Autodesk Fusion 360 part; units mm, degrees
note: some values were not read from the file. Set by a fixed rule: the direction of a hole.
(part 7 of 10)
  arc A53 (93.84, 10.795) -> (97.04, 10.795) centre (95.44, 10.795) ccw
  arc A54 (97.04, 15.875) -> (93.84, 15.875) centre (95.44, 15.875) ccw
  arc A55 (93.84, 15.875) -> (97.04, 15.875) centre (95.44, 15.875) ccw
  arc A56 (6.731, 3.81) -> (0.889, 3.81) centre (3.81, 3.81) ccw
  arc A57 (0.889, 3.81) -> (6.731, 3.81) centre (3.81, 3.81) ccw
  arc A58 (2.31, 3.81) -> (5.31, 3.81) centre (3.81, 3.81) ccw
  arc A59 (5.31, 3.81) -> (2.31, 3.81) centre (3.81, 3.81) ccw
  arc A60 (99.441, 76.2) -> (93.599, 76.2) centre (96.52, 76.2) ccw
  arc A61 (93.599, 76.2) -> (99.441, 76.2) centre (96.52, 76.2) ccw
  arc A62 (95.02, 76.2) -> (98.02, 76.2) centre (96.52, 76.2) ccw
  arc A63 (98.02, 76.2) -> (95.02, 76.2) centre (96.52, 76.2) ccw
  arc A64 (0.889, 76.2) -> (6.731, 76.2) centre (3.81, 76.2) ccw
  arc A65 (6.731, 76.2) -> (0.889, 76.2) centre (3.81, 76.2) ccw
  arc A66 (5.31, 76.2) -> (2.31, 76.2) centre (3.81, 76.2) ccw
  arc A67 (2.31, 76.2) -> (5.31, 76.2) centre (3.81, 76.2) ccw
  arc A68 (99.441, 3.81) -> (93.599, 3.81) centre (96.52, 3.81) ccw
  arc A69 (93.599, 3.81) -> (99.441, 3.81) centre (96.52, 3.81) ccw
  arc A70 (98.02, 3.81) -> (95.02, 3.81) centre (96.52, 3.81) ccw
  arc A71 (95.02, 3.81) -> (98.02, 3.81) centre (96.52, 3.81) ccw
  line L5675 (36.52, 58.32) -> (36.52, 71.07)
  line L5676 (36.52, 71.07) -> (4.02, 71.07)
  line L5677 (4.02, 71.07) -> (4.02, 58.32)
  line L5678 (4.02, 58.32) -> (36.52, 58.32)
  line L5679 (63.81, 71.22) -> (63.81, 58.47)
  line L5680 (63.81, 58.47) -> (96.31, 58.47)
  line L5681 (96.31, 58.47) -> (96.31, 71.22)
  line L5682 (96.31, 71.22) -> (63.81, 71.22)
  line L5683 (10.143, 54.229) -> (1.143, 54.229)
  line L5684 (1.143, 54.229) -> (1.143, 32.229)
  line L5685 (1.143, 32.229) -> (10.143, 32.229)
  line L5686 (10.143, 32.229) -> (10.143, 54.229)
  line L5687 (22.843, 54.229) -> (13.843, 54.229)
  line L5688 (13.843, 54.229) -> (13.843, 32.229)
  line L5689 (13.843, 32.229) -> (22.843, 32.229)
  line L5690 (22.843, 32.229) -> (22.843, 54.229)
  line L5691 (35.543, 54.229) -> (26.543, 54.229)
  line L5692 (26.543, 54.229) -> (26.543, 32.229)
  line L5693 (26.543, 32.229) -> (35.543, 32.229)
  line L5694 (35.543, 32.229) -> (35.543, 54.229)
  line L5695 (48.243, 54.229) -> (39.243, 54.229)
  line L5696 (39.243, 54.229) -> (39.243, 32.229)
  line L5697 (39.243, 32.229) -> (48.243, 32.229)
  line L5698 (48.243, 32.229) -> (48.243, 54.229)
  line L5699 (61.578, 54.229) -> (52.578, 54.229)
  line L5700 (52.578, 54.229) -> (52.578, 32.229)
  line L5701 (52.578, 32.229) -> (61.578, 32.229)
  line L5702 (61.578, 32.229) -> (61.578, 54.229)
  line L5703 (74.278, 54.229) -> (65.278, 54.229)
  line L5704 (65.278, 54.229) -> (65.278, 32.229)
  line L5705 (65.278, 32.229) -> (74.278, 32.229)
  line L5706 (74.278, 32.229) -> (74.278, 54.229)
  line L5707 (86.978, 54.229) -> (77.978, 54.229)
  line L5708 (77.978, 54.229) -> (77.978, 32.229)
  line L5709 (77.978, 32.229) -> (86.978, 32.229)
  line L5710 (86.978, 32.229) -> (86.978, 54.229)
  line L5711 (99.043, 54.229) -> (90.043, 54.229)
  line L5712 (90.043, 54.229) -> (90.043, 32.229)
  line L5713 (90.043, 32.229) -> (99.043, 32.229)
  line L5714 (99.043, 32.229) -> (99.043, 54.229)
  line L5715 (50.8, 79.375) -> (50.8, 71.375)
  line L5716 (55.88, 79.375) -> (50.8, 79.375)
  line L5717 (50.8, 79.375) -> (45.72, 79.375)
  line L5718 (45.72, 79.375) -> (45.72, 78.74)
  line L5719 (45.72, 78.74) -> (45.72, 72.0725)
  line L5720 (45.72, 72.0725) -> (45.72, 71.375)
  line L5721 (45.72, 71.375) -> (50.8, 71.375)
  line L5722 (50.8, 71.375) -> (55.88, 71.375)
  line L5723 (55.88, 71.375) -> (55.88, 72.0725)
  line L5724 (55.88, 72.0725) -> (55.88, 72.263)
  line L5725 (55.88, 72.263) -> (55.88, 73.025)
  line L5726 (55.88, 73.025) -> (55.88, 78.74)
  line L5727 (55.88, 78.74) -> (55.88, 79.375)
  line L5728 (55.88, 72.0725) -> (45.72, 72.0725)
  line L5729 (55.88, 72.263) -> (56.388, 71.755)
  line L5730 (56.388, 71.755) -> (56.388, 73.533)
  line L5731 (56.388, 73.533) -> (55.88, 73.025)
  line L5732 (55.88, 78.74) -> (45.72, 78.74)
  line L5733 (0.635, 13.335) -> (8.635, 13.335)
  line L5734 (0.635, 18.415) -> (0.635, 13.335)
  line L5735 (0.635, 13.335) -> (0.635, 8.255)
  line L5736 (0.635, 8.255) -> (1.27, 8.255)
  line L5737 (1.27, 8.255) -> (7.9375, 8.255)
  line L5738 (7.9375, 8.255) -> (8.635, 8.255)
  line L5739 (8.635, 8.255) -> (8.635, 13.335)
  line L5740 (8.635, 13.335) -> (8.635, 18.415)
  line L5741 (8.635, 18.415) -> (7.9375, 18.415)
  line L5742 (7.9375, 18.415) -> (7.747, 18.415)
  line L5743 (7.747, 18.415) -> (6.985, 18.415)
  line L5744 (6.985, 18.415) -> (1.27, 18.415)
  line L5745 (1.27, 18.415) -> (0.635, 18.415)
  line L5746 (7.9375, 18.415) -> (7.9375, 8.255)
  line L5747 (7.747, 18.415) -> (8.255, 18.923)
  line L5748 (8.255, 18.923) -> (6.477, 18.923)
  line L5749 (6.477, 18.923) -> (6.985, 18.415)
  line L5750 (1.27, 18.415) -> (1.27, 8.255)
  line L5751 (18.415, 8.89) -> (18.415, 0.89)
  line L5752 (23.495, 8.89) -> (18.415, 8.89)
  line L5753 (18.415, 8.89) -> (13.335, 8.89)
  line L5754 (13.335, 8.89) -> (13.335, 8.255)
  line L5755 (13.335, 8.255) -> (13.335, 1.5875)
  line L5756 (13.335, 1.5875) -> (13.335, 0.89)
  line L5757 (13.335, 0.89) -> (18.415, 0.89)
  line L5758 (18.415, 0.89) -> (23.495, 0.89)
  line L5759 (23.495, 0.89) -> (23.495, 1.5875)
  line L5760 (23.495, 1.5875) -> (23.495, 1.778)
  line L5761 (23.495, 1.778) -> (23.495, 2.54)
  line L5762 (23.495, 2.54) -> (23.495, 8.255)
  line L5763 (23.495, 8.255) -> (23.495, 8.89)
  line L5764 (23.495, 1.5875) -> (13.335, 1.5875)
  line L5765 (23.495, 1.778) -> (24.003, 1.27)
  line L5766 (24.003, 1.27) -> (24.003, 3.048)
  line L5767 (24.003, 3.048) -> (23.495, 2.54)
  line L5768 (23.495, 8.255) -> (13.335, 8.255)
  line L5769 (31.115, 8.89) -> (31.115, 0.89)
  line L5770 (36.195, 8.89) -> (31.115, 8.89)
  line L5771 (31.115, 8.89) -> (26.035, 8.89)
  line L5772 (26.035, 8.89) -> (26.035, 8.255)
  line L5773 (26.035, 8.255) -> (26.035, 1.5875)
  line L5774 (26.035, 1.5875) -> (26.035, 0.89)
  line L5775 (26.035, 0.89) -> (31.115, 0.89)
  line L5776 (31.115, 0.89) -> (36.195, 0.89)
  line L5777 (36.195, 0.89) -> (36.195, 1.5875)
  line L5778 (36.195, 1.5875) -> (36.195, 1.778)
  line L5779 (36.195, 1.778) -> (36.195, 2.54)
  line L5780 (36.195, 2.54) -> (36.195, 8.255)
  line L5781 (36.195, 8.255) -> (36.195, 8.89)
  line L5782 (36.195, 1.5875) -> (26.035, 1.5875)
  line L5783 (36.195, 1.778) -> (36.703, 1.27)
  line L5784 (36.703, 1.27) -> (36.703, 3.048)
  line L5785 (36.703, 3.048) -> (36.195, 2.54)
  line L5786 (36.195, 8.255) -> (26.035, 8.255)
  line L5787 (43.815, 8.89) -> (43.815, 0.89)
  line L5788 (48.895, 8.89) -> (43.815, 8.89)
  line L5789 (43.815, 8.89) -> (38.735, 8.89)
  line L5790 (38.735, 8.89) -> (38.735, 8.255)
  line L5791 (38.735, 8.255) -> (38.735, 1.5875)
  line L5792 (38.735, 1.5875) -> (38.735, 0.89)
  line L5793 (38.735, 0.89) -> (43.815, 0.89)
  line L5794 (43.815, 0.89) -> (48.895, 0.89)
  line L5795 (48.895, 0.89) -> (48.895, 1.5875)
  line L5796 (48.895, 1.5875) -> (48.895, 1.778)
  line L5797 (48.895, 1.778) -> (48.895, 2.54)
  line L5798 (48.895, 2.54) -> (48.895, 8.255)
  line L5799 (48.895, 8.255) -> (48.895, 8.89)
  line L5800 (48.895, 1.5875) -> (38.735, 1.5875)
  line L5801 (48.895, 1.778) -> (49.403, 1.27)
  line L5802 (49.403, 1.27) -> (49.403, 3.048)
  line L5803 (49.403, 3.048) -> (48.895, 2.54)
  line L5804 (48.895, 8.255) -> (38.735, 8.255)
  line L5805 (57.15, 8.89) -> (57.15, 0.89)
  line L5806 (62.23, 8.89) -> (57.15, 8.89)
  line L5807 (57.15, 8.89) -> (52.07, 8.89)
  line L5808 (52.07, 8.89) -> (52.07, 8.255)
  line L5809 (52.07, 8.255) -> (52.07, 1.5875)
  line L5810 (52.07, 1.5875) -> (52.07, 0.89)
  line L5811 (52.07, 0.89) -> (57.15, 0.89)
  line L5812 (57.15, 0.89) -> (62.23, 0.89)
  line L5813 (62.23, 0.89) -> (62.23, 1.5875)
  line L5814 (62.23, 1.5875) -> (62.23, 1.778)
  line L5815 (62.23, 1.778) -> (62.23, 2.54)
  line L5816 (62.23, 2.54) -> (62.23, 8.255)
  line L5817 (62.23, 8.255) -> (62.23, 8.89)
  line L5818 (62.23, 1.5875) -> (52.07, 1.5875)
  line L5819 (62.23, 1.778) -> (62.738, 1.27)
  line L5820 (62.738, 1.27) -> (62.738, 3.048)
  line L5821 (62.738, 3.048) -> (62.23, 2.54)
  line L5822 (62.23, 8.255) -> (52.07, 8.255)
  line L5823 (69.85, 8.89) -> (69.85, 0.89)
  line L5824 (74.93, 8.89) -> (69.85, 8.89)
  line L5825 (69.85, 8.89) -> (64.77, 8.89)
  line L5826 (64.77, 8.89) -> (64.77, 8.255)
  line L5827 (64.77, 8.255) -> (64.77, 1.5875)
  line L5828 (64.77, 1.5875) -> (64.77, 0.89)
  line L5829 (64.77, 0.89) -> (69.85, 0.89)
  line L5830 (69.85, 0.89) -> (74.93, 0.89)
  line L5831 (74.93, 0.89) -> (74.93, 1.5875)
  line L5832 (74.93, 1.5875) -> (74.93, 1.778)
  line L5833 (74.93, 1.778) -> (74.93, 2.54)
  line L5834 (74.93, 2.54) -> (74.93, 8.255)
  line L5835 (74.93, 8.255) -> (74.93, 8.89)
  line L5836 (74.93, 1.5875) -> (64.77, 1.5875)
  line L5837 (74.93, 1.778) -> (75.438, 1.27)
  line L5838 (75.438, 1.27) -> (75.438, 3.048)
  line L5839 (75.438, 3.048) -> (74.93, 2.54)
  line L5840 (74.93, 8.255) -> (64.77, 8.255)
  line L5841 (82.55, 8.89) -> (82.55, 0.89)
  line L5842 (87.63, 8.89) -> (82.55, 8.89)
  line L5843 (82.55, 8.89) -> (77.47, 8.89)
  line L5844 (77.47, 8.89) -> (77.47, 8.255)
  line L5845 (77.47, 8.255) -> (77.47, 1.5875)
  line L5846 (77.47, 1.5875) -> (77.47, 0.89)
  line L5847 (77.47, 0.89) -> (82.55, 0.89)
  line L5848 (82.55, 0.89) -> (87.63, 0.89)
  line L5849 (87.63, 0.89) -> (87.63, 1.5875)
  line L5850 (87.63, 1.5875) -> (87.63, 1.778)
  line L5851 (87.63, 1.778) -> (87.63, 2.54)
  line L5852 (87.63, 2.54) -> (87.63, 8.255)
  line L5853 (87.63, 8.255) -> (87.63, 8.89)
  line L5854 (87.63, 1.5875) -> (77.47, 1.5875)
  line L5855 (87.63, 1.778) -> (88.138, 1.27)
  line L5856 (88.138, 1.27) -> (88.138, 3.048)
  line L5857 (88.138, 3.048) -> (87.63, 2.54)
  line L5858 (87.63, 8.255) -> (77.47, 8.255)
  line L5859 (91.44, 13.335) -> (99.44, 13.335)
  line L5860 (91.44, 18.415) -> (91.44, 13.335)
  line L5861 (91.44, 13.335) -> (91.44, 8.255)
  line L5862 (91.44, 8.255) -> (92.075, 8.255)
  line L5863 (92.075, 8.255) -> (98.7425, 8.255)
  line L5864 (98.7425, 8.255) -> (99.44, 8.255)
  line L5865 (99.44, 8.255) -> (99.44, 13.335)
  line L5866 (99.44, 13.335) -> (99.44, 18.415)
  line L5867 (99.44, 18.415) -> (98.7425, 18.415)
  line L5868 (98.7425, 18.415) -> (98.552, 18.415)
  line L5869 (98.552, 18.415) -> (97.79, 18.415)
  line L5870 (97.79, 18.415) -> (92.075, 18.415)
  line L5871 (92.075, 18.415) -> (91.44, 18.415)
  line L5872 (98.7425, 18.415) -> (98.7425, 8.255)
  line L5873 (98.552, 18.415) -> (99.06, 18.923)
  line L5874 (99.06, 18.923) -> (97.282, 18.923)
  line L5875 (97.282, 18.923) -> (97.79, 18.415)
  line L5876 (92.075, 18.415) -> (92.075, 8.255)
  arc A72 (22.86, 78.359) -> (24.1001, 77.7208) centre (22.86, 76.835) cw
  arc A73 (21.6408, 77.7494) -> (22.86, 78.359) centre (22.86, 76.835) cw
  arc A74 (22.86, 75.311) -> (24.063, 75.8994) centre (22.86, 76.835) ccw
  arc A75 (21.657, 75.8994) -> (22.86, 75.311) centre (22.86, 76.835) ccw
  arc A76 (22.86, 78.867) -> (24.421, 78.1359) centre (22.86, 76.835) cw
  arc A77 (21.0671, 77.7912) -> (22.86, 78.867) centre (22.8601, 76.835) cw
  arc A78 (22.86, 74.803) -> (24.4112, 75.5224) centre (22.86, 76.835) ccw
  arc A79 (21.0957, 75.8268) -> (22.86, 74.803) centre (22.8599, 76.835) ccw
  arc A80 (77.47, 74.676) -> (76.2299, 75.3142) centre (77.47, 76.2) cw
  arc A81 (78.6892, 75.2856) -> (77.47, 74.676) centre (77.47, 76.2) cw
  arc A82 (77.47, 77.724) -> (76.267, 77.1356) centre (77.47, 76.2) ccw
  arc A83 (78.673, 77.1356) -> (77.47, 77.724) centre (77.47, 76.2) ccw
  arc A84 (77.47, 74.168) -> (75.909, 74.8991) centre (77.47, 76.2) cw
  arc A85 (79.2629, 75.2438) -> (77.47, 74.168) centre (77.4699, 76.2) cw
  arc A86 (77.47, 78.232) -> (75.9188, 77.5126) centre (77.47, 76.2) ccw
  arc A87 (79.2343, 77.2082) -> (77.47, 78.232) centre (77.4701, 76.2) ccw
  arc A88 (11.43, 18.034) -> (12.6701, 17.3958) centre (11.43, 16.51) cw
  arc A89 (10.2108, 17.4244) -> (11.43, 18.034) centre (11.43, 16.51) cw
  arc A90 (11.43, 14.986) -> (12.633, 15.5744) centre (11.43, 16.51) ccw
  arc A91 (10.227, 15.5744) -> (11.43, 14.986) centre (11.43, 16.51) ccw
  arc A92 (11.43, 18.542) -> (12.991, 17.8109) centre (11.43, 16.51) cw
  arc A93 (9.6371, 17.4662) -> (11.43, 18.542) centre (11.4301, 16.51) cw
  arc A94 (11.43, 14.478) -> (12.9812, 15.1974) centre (11.43, 16.51) ccw
  arc A95 (9.6657, 15.5018) -> (11.43, 14.478) centre (11.4299, 16.51) ccw
  arc A96 (77.47, 14.986) -> (76.2299, 15.6242) centre (77.47, 16.51) cw
  arc A97 (78.6892, 15.5956) -> (77.47, 14.986) centre (77.47, 16.51) cw
  arc A98 (77.47, 18.034) -> (76.267, 17.4456) centre (77.47, 16.51) ccw
  arc A99 (78.673, 17.4456) -> (77.47, 18.034) centre (77.47, 16.51) ccw
  arc A100 (77.47, 14.478) -> (75.909, 15.2091) centre (77.47, 16.51) cw
  arc A101 (79.2629, 15.5538) -> (77.47, 14.478) centre (77.4699, 16.51) cw
  arc A102 (77.47, 18.542) -> (75.9188, 17.8226) centre (77.47, 16.51) ccw
  arc A103 (79.2343, 17.5182) -> (77.47, 18.542) centre (77.4701, 16.51) ccw
  arc A104 (66.04, 14.986) -> (64.7999, 15.6242) centre (66.04, 16.51) cw
  arc A105 (67.2592, 15.5956) -> (66.04, 14.986) centre (66.04, 16.51) cw
  arc A106 (66.04, 18.034) -> (64.837, 17.4456) centre (66.04, 16.51) ccw
  arc A107 (67.243, 17.4456) -> (66.04, 18.034) centre (66.04, 16.51) ccw
  arc A108 (66.04, 14.478) -> (64.479, 15.2091) centre (66.04, 16.51) cw
  arc A109 (67.8329, 15.5538) -> (66.04, 14.478) centre (66.0399, 16.51) cw
  arc A110 (66.04, 18.542) -> (64.4888, 17.8226) centre (66.04, 16.51) ccw
  arc A111 (67.8043, 17.5182) -> (66.04, 18.542) centre (66.0401, 16.51) ccw
  arc A112 (55.88, 14.986) -> (54.6399, 15.6242) centre (55.88, 16.51) cw
  arc A113 (57.0992, 15.5956) -> (55.88, 14.986) centre (55.88, 16.51) cw
  arc A114 (55.88, 18.034) -> (54.677, 17.4456) centre (55.88, 16.51) ccw
  arc A115 (57.083, 17.4456) -> (55.88, 18.034) centre (55.88, 16.51) ccw
  arc A116 (55.88, 14.478) -> (54.319, 15.2091) centre (55.88, 16.51) cw
  arc A117 (57.6729, 15.5538) -> (55.88, 14.478) centre (55.8799, 16.51) cw
  arc A118 (55.88, 18.542) -> (54.3288, 17.8226) centre (55.88, 16.51) ccw
  arc A119 (57.6443, 17.5182) -> (55.88, 18.542) centre (55.8801, 16.51) ccw
  arc A120 (47.625, 18.034) -> (48.8651, 17.3958) centre (47.625, 16.51) cw
  arc A121 (46.4058, 17.4244) -> (47.625, 18.034) centre (47.625, 16.51) cw
  arc A122 (47.625, 14.986) -> (48.828, 15.5744) centre (47.625, 16.51) ccw
  arc A123 (46.422, 15.5744) -> (47.625, 14.986) centre (47.625, 16.51) ccw
  arc A124 (47.625, 18.542) -> (49.186, 17.8109) centre (47.625, 16.51) cw
  arc A125 (45.8321, 17.4662) -> (47.625, 18.542) centre (47.6251, 16.51) cw
  arc A126 (47.625, 14.478) -> (49.1762, 15.1974) centre (47.625, 16.51) ccw
  arc A127 (45.8607, 15.5018) -> (47.625, 14.478) centre (47.6249, 16.51) ccw
  arc A128 (36.83, 18.034) -> (38.0701, 17.3958) centre (36.83, 16.51) cw
  arc A129 (35.6108, 17.4244) -> (36.83, 18.034) centre (36.83, 16.51) cw
  arc A130 (36.83, 14.986) -> (38.033, 15.5744) centre (36.83, 16.51) ccw
  arc A131 (35.627, 15.5744) -> (36.83, 14.986) centre (36.83, 16.51) ccw
  arc A132 (36.83, 18.542) -> (38.391, 17.8109) centre (36.83, 16.51) cw
  arc A133 (35.0371, 17.4662) -> (36.83, 18.542) centre (36.8301, 16.51) cw
  arc A134 (36.83, 14.478) -> (38.3812, 15.1974) centre (36.83, 16.51) ccw
  arc A135 (35.0657, 15.5018) -> (36.83, 14.478) centre (36.8299, 16.51) ccw
  arc A136 (24.13, 18.034) -> (25.3701, 17.3958) centre (24.13, 16.51) cw
  arc A137 (22.9108, 17.4244) -> (24.13, 18.034) centre (24.13, 16.51) cw
  arc A138 (24.13, 14.986) -> (25.333, 15.5744) centre (24.13, 16.51) ccw
  arc A139 (22.927, 15.5744) -> (24.13, 14.986) centre (24.13, 16.51) ccw
  arc A140 (24.13, 18.542) -> (25.691, 17.8109) centre (24.13, 16.51) cw
  arc A141 (22.3371, 17.4662) -> (24.13, 18.542) centre (24.1301, 16.51) cw
  arc A142 (24.13, 14.478) -> (25.6812, 15.1974) centre (24.13, 16.51) ccw
  arc A143 (22.3657, 15.5018) -> (24.13, 14.478) centre (24.1299, 16.51) ccw
  arc A144 (88.9, 14.986) -> (87.6599, 15.6242) centre (88.9, 16.51) cw
  arc A145 (90.1192, 15.5956) -> (88.9, 14.986) centre (88.9, 16.51) cw
  arc A146 (88.9, 18.034) -> (87.697, 17.4456) centre (88.9, 16.51) ccw
  arc A147 (90.103, 17.4456) -> (88.9, 18.034) centre (88.9, 16.51) ccw
  arc A148 (88.9, 14.478) -> (87.339, 15.2091) centre (88.9, 16.51) cw
  arc A149 (90.6929, 15.5538) -> (88.9, 14.478) centre (88.8999, 16.51) cw
  arc A150 (88.9, 18.542) -> (87.3488, 17.8226) centre (88.9, 16.51) ccw
  arc A151 (90.6643, 17.5182) -> (88.9, 18.542) centre (88.9001, 16.51) ccw
  arc A152 (17.145, 75.946) -> (16.891, 75.692) centre (16.891, 75.946) cw
  arc A153 (17.145, 77.724) -> (16.891, 77.978) centre (16.891, 77.724) ccw
  arc A154 (11.049, 77.978) -> (10.795, 77.724) centre (11.049, 77.724) ccw
  arc A155 (11.049, 75.692) -> (10.795, 75.946) centre (11.049, 75.946) cw
  line L5877 (17.145, 77.724) -> (17.145, 75.946)
  line L5878 (16.891, 75.692) -> (16.51, 75.692)
  line L5879 (16.383, 75.819) -> (16.51, 75.692)
  line L5880 (16.891, 77.978) -> (16.51, 77.978)
  line L5881 (16.383, 77.851) -> (16.51, 77.978)
  line L5882 (11.557, 75.819) -> (11.43, 75.692)
  line L5883 (11.557, 75.819) -> (16.383, 75.819)
  line L5884 (11.557, 77.851) -> (11.43, 77.978)
  line L5885 (11.557, 77.851) -> (16.383, 77.851)
  line L5886 (11.049, 75.692) -> (11.43, 75.692)
  line L5887 (11.049, 77.978) -> (11.43, 77.978)
  line L5888 (10.795, 77.724) -> (10.795, 75.946)
  arc A156 (83.185, 77.089) -> (83.439, 77.343) centre (83.439, 77.089) cw
  arc A157 (83.185, 75.311) -> (83.439, 75.057) centre (83.439, 75.311) ccw
  arc A158 (89.281, 75.057) -> (89.535, 75.311) centre (89.281, 75.311) ccw
  arc A159 (89.281, 77.343) -> (89.535, 77.089) centre (89.281, 77.089) cw
  line L5889 (83.185, 75.311) -> (83.185, 77.089)
  line L5890 (83.439, 77.343) -> (83.82, 77.343)
  line L5891 (83.947, 77.216) -> (83.82, 77.343)
  line L5892 (83.439, 75.057) -> (83.82, 75.057)
  line L5893 (83.947, 75.184) -> (83.82, 75.057)
  line L5894 (88.773, 77.216) -> (88.9, 77.343)
  line L5895 (88.773, 77.216) -> (83.947, 77.216)
  line L5896 (88.773, 75.184) -> (88.9, 75.057)
  line L5897 (88.773, 75.184) -> (83.947, 75.184)
  line L5898 (89.281, 77.343) -> (88.9, 77.343)
  line L5899 (89.281, 75.057) -> (88.9, 75.057)
  line L5900 (89.535, 75.311) -> (89.535, 77.089)
  arc A160 (9.271, 22.225) -> (9.017, 22.479) centre (9.271, 22.479) cw
  arc A161 (11.049, 22.225) -> (11.303, 22.479) centre (11.049, 22.479) ccw
  arc A162 (11.303, 28.321) -> (11.049, 28.575) centre (11.049, 28.321) ccw
  arc A163 (9.017, 28.321) -> (9.271, 28.575) centre (9.271, 28.321) cw
  line L5901 (11.049, 22.225) -> (9.271, 22.225)
  line L5902 (9.017, 22.479) -> (9.017, 22.86)
  line L5903 (9.144, 22.987) -> (9.017, 22.86)
  line L5904 (11.303, 22.479) -> (11.303, 22.86)
  line L5905 (11.176, 22.987) -> (11.303, 22.86)
  line L5906 (9.144, 27.813) -> (9.017, 27.94)
  line L5907 (9.144, 27.813) -> (9.144, 22.987)
  line L5908 (11.176, 27.813) -> (11.303, 27.94)
  line L5909 (11.176, 27.813) -> (11.176, 22.987)
  line L5910 (9.017, 28.321) -> (9.017, 27.94)
  line L5911 (11.303, 28.321) -> (11.303, 27.94)
  line L5912 (11.049, 28.575) -> (9.271, 28.575)
  arc A164 (21.971, 22.225) -> (21.717, 22.479) centre (21.971, 22.479) cw
  arc A165 (23.749, 22.225) -> (24.003, 22.479) centre (23.749, 22.479) ccw
  arc A166 (24.003, 28.321) -> (23.749, 28.575) centre (23.749, 28.321) ccw
  arc A167 (21.717, 28.321) -> (21.971, 28.575) centre (21.971, 28.321) cw
  line L5913 (23.749, 22.225) -> (21.971, 22.225)
  line L5914 (21.717, 22.479) -> (21.717, 22.86)
  line L5915 (21.844, 22.987) -> (21.717, 22.86)
  line L5916 (24.003, 22.479) -> (24.003, 22.86)
  line L5917 (23.876, 22.987) -> (24.003, 22.86)
  line L5918 (21.844, 27.813) -> (21.717, 27.94)
  line L5919 (21.844, 27.813) -> (21.844, 22.987)
  line L5920 (23.876, 27.813) -> (24.003, 27.94)
  line L5921 (23.876, 27.813) -> (23.876, 22.987)
  line L5922 (21.717, 28.321) -> (21.717, 27.94)
  line L5923 (24.003, 28.321) -> (24.003, 27.94)
  line L5924 (23.749, 28.575) -> (21.971, 28.575)
  arc A168 (34.671, 22.225) -> (34.417, 22.479) centre (34.671, 22.479) cw
  arc A169 (36.449, 22.225) -> (36.703, 22.479) centre (36.449, 22.479) ccw
  arc A170 (36.703, 28.321) -> (36.449, 28.575) centre (36.449, 28.321) ccw
  arc A171 (34.417, 28.321) -> (34.671, 28.575) centre (34.671, 28.321) cw
  line L5925 (36.449, 22.225) -> (34.671, 22.225)
  line L5926 (34.417, 22.479) -> (34.417, 22.86)
  line L5927 (34.544, 22.987) -> (34.417, 22.86)
  line L5928 (36.703, 22.479) -> (36.703, 22.86)
  line L5929 (36.576, 22.987) -> (36.703, 22.86)
  line L5930 (34.544, 27.813) -> (34.417, 27.94)
  line L5931 (34.544, 27.813) -> (34.544, 22.987)
  line L5932 (36.576, 27.813) -> (36.703, 27.94)
  line L5933 (36.576, 27.813) -> (36.576, 22.987)
  line L5934 (34.417, 28.321) -> (34.417, 27.94)
  line L5935 (36.703, 28.321) -> (36.703, 27.94)
  line L5936 (36.449, 28.575) -> (34.671, 28.575)
  arc A172 (47.371, 22.225) -> (47.117, 22.479) centre (47.371, 22.479) cw
  arc A173 (49.149, 22.225) -> (49.403, 22.479) centre (49.149, 22.479) ccw
  arc A174 (49.403, 28.321) -> (49.149, 28.575) centre (49.149, 28.321) ccw
  arc A175 (47.117, 28.321) -> (47.371, 28.575) centre (47.371, 28.321) cw
  line L5937 (49.149, 22.225) -> (47.371, 22.225)
  line L5938 (47.117, 22.479) -> (47.117, 22.86)
  line L5939 (47.244, 22.987) -> (47.117, 22.86)
  line L5940 (49.403, 22.479) -> (49.403, 22.86)
  line L5941 (49.276, 22.987) -> (49.403, 22.86)
  line L5942 (47.244, 27.813) -> (47.117, 27.94)
  line L5943 (47.244, 27.813) -> (47.244, 22.987)
  line L5944 (49.276, 27.813) -> (49.403, 27.94)
  line L5945 (49.276, 27.813) -> (49.276, 22.987)
  line L5946 (47.117, 28.321) -> (47.117, 27.94)
  line L5947 (49.403, 28.321) -> (49.403, 27.94)
  line L5948 (49.149, 28.575) -> (47.371, 28.575)
  arc A176 (52.451, 22.225) -> (52.197, 22.479) centre (52.451, 22.479) cw
  arc A177 (54.229, 22.225) -> (54.483, 22.479) centre (54.229, 22.479) ccw
  arc A178 (54.483, 28.321) -> (54.229, 28.575) centre (54.229, 28.321) ccw
  arc A179 (52.197, 28.321) -> (52.451, 28.575) centre (52.451, 28.321) cw
  line L5949 (54.229, 22.225) -> (52.451, 22.225)
  line L5950 (52.197, 22.479) -> (52.197, 22.86)
  line L5951 (52.324, 22.987) -> (52.197, 22.86)
  line L5952 (54.483, 22.479) -> (54.483, 22.86)
  line L5953 (54.356, 22.987) -> (54.483, 22.86)
  line L5954 (52.324, 27.813) -> (52.197, 27.94)
  line L5955 (52.324, 27.813) -> (52.324, 22.987)
  line L5956 (54.356, 27.813) -> (54.483, 27.94)
  line L5957 (54.356, 27.813) -> (54.356, 22.987)
  line L5958 (52.197, 28.321) -> (52.197, 27.94)
  line L5959 (54.483, 28.321) -> (54.483, 27.94)
  line L5960 (54.229, 28.575) -> (52.451, 28.575)
  arc A180 (66.421, 22.225) -> (66.167, 22.479) centre (66.421, 22.479) cw
  arc A181 (68.199, 22.225) -> (68.453, 22.479) centre (68.199, 22.479) ccw
  arc A182 (68.453, 28.321) -> (68.199, 28.575) centre (68.199, 28.321) ccw
  arc A183 (66.167, 28.321) -> (66.421, 28.575) centre (66.421, 28.321) cw
  line L5961 (68.199, 22.225) -> (66.421, 22.225)
  line L5962 (66.167, 22.479) -> (66.167, 22.86)
  line L5963 (66.294, 22.987) -> (66.167, 22.86)
  line L5964 (68.453, 22.479) -> (68.453, 22.86)
  line L5965 (68.326, 22.987) -> (68.453, 22.86)
  line L5966 (66.294, 27.813) -> (66.167, 27.94)
  line L5967 (66.294, 27.813) -> (66.294, 22.987)
  line L5968 (68.326, 27.813) -> (68.453, 27.94)
  line L5969 (68.326, 27.813) -> (68.326, 22.987)
  line L5970 (66.167, 28.321) -> (66.167, 27.94)
  line L5971 (68.453, 28.321) -> (68.453, 27.94)
  line L5972 (68.199, 28.575) -> (66.421, 28.575)
  arc A184 (77.851, 22.225) -> (77.597, 22.479) centre (77.851, 22.479) cw
  arc A185 (79.629, 22.225) -> (79.883, 22.479) centre (79.629, 22.479) ccw
  arc A186 (79.883, 28.321) -> (79.629, 28.575) centre (79.629, 28.321) ccw
  arc A187 (77.597, 28.321) -> (77.851, 28.575) centre (77.851, 28.321) cw
  line L5973 (79.629, 22.225) -> (77.851, 22.225)
  line L5974 (77.597, 22.479) -> (77.597, 22.86)
  line L5975 (77.724, 22.987) -> (77.597, 22.86)
  line L5976 (79.883, 22.479) -> (79.883, 22.86)
  line L5977 (79.756, 22.987) -> (79.883, 22.86)
  line L5978 (77.724, 27.813) -> (77.597, 27.94)
  line L5979 (77.724, 27.813) -> (77.724, 22.987)
  line L5980 (79.756, 27.813) -> (79.883, 27.94)
  line L5981 (79.756, 27.813) -> (79.756, 22.987)
  line L5982 (77.597, 28.321) -> (77.597, 27.94)
  line L5983 (79.883, 28.321) -> (79.883, 27.94)
  line L5984 (79.629, 28.575) -> (77.851, 28.575)
  arc A188 (89.281, 22.225) -> (89.027, 22.479) centre (89.281, 22.479) cw
  arc A189 (91.059, 22.225) -> (91.313, 22.479) centre (91.059, 22.479) ccw
  arc A190 (91.313, 28.321) -> (91.059, 28.575) centre (91.059, 28.321) ccw
  arc A191 (89.027, 28.321) -> (89.281, 28.575) centre (89.281, 28.321) cw
  line L5985 (91.059, 22.225) -> (89.281, 22.225)
  line L5986 (89.027, 22.479) -> (89.027, 22.86)
  line L5987 (89.154, 22.987) -> (89.027, 22.86)
  line L5988 (91.313, 22.479) -> (91.313, 22.86)
  line L5989 (91.186, 22.987) -> (91.313, 22.86)
  line L5990 (89.154, 27.813) -> (89.027, 27.94)
  line L5991 (89.154, 27.813) -> (89.154, 22.987)
  line L5992 (91.186, 27.813) -> (91.313, 27.94)
  line L5993 (91.186, 27.813) -> (91.186, 22.987)
  line L5994 (89.027, 28.321) -> (89.027, 27.94)
  line L5995 (91.313, 28.321) -> (91.313, 27.94)
  line L5996 (91.059, 28.575) -> (89.281, 28.575)
  arc A192 (36.9326, 76.3477) -> (37.2918, 76.3477) centre (37.1122, 76.1681) cw
  arc A193 (35.6753, 75.0905) -> (35.6753, 74.7312) centre (35.8549, 74.9109) ccw
  arc A194 (39.8062, 70.6003) -> (40.1655, 70.6003) centre (39.9859, 70.7799) ccw
  arc A195 (41.4227, 72.2168) -> (41.4227, 71.8576) centre (41.2431, 72.0372) cw
  line L5997 (35.6753, 75.0905) -> (36.9326, 76.3477)
  line L5998 (37.2918, 76.3477) -> (37.5612, 76.0783)
  line L5999 (37.5612, 75.8987) -> (37.5612, 76.0783)
  line L6000 (35.6753, 74.7312) -> (35.9447, 74.4618)
  line L6001 (36.1243, 74.4618) -> (35.9447, 74.4618)
  line L6002 (40.9737, 72.4862) -> (41.1533, 72.4862)
  line L6003 (40.9737, 72.4862) -> (37.5612, 75.8987)
  line L6004 (39.5368, 71.0493) -> (39.5368, 70.8697)
  line L6005 (39.5368, 71.0493) -> (36.1243, 74.4618)
  line L6006 (41.4227, 72.2168) -> (41.1533, 72.4862)
  line L6007 (39.8062, 70.6003) -> (39.5368, 70.8697)
  line L6008 (40.1655, 70.6003) -> (41.4227, 71.8576)
  arc A196 (27.94, 75.311) -> (26.6999, 75.9492) centre (27.94, 76.835) cw
  arc A197 (29.1592, 75.9206) -> (27.94, 75.311) centre (27.94, 76.835) cw
  arc A198 (27.94, 78.359) -> (26.737, 77.7706) centre (27.94, 76.835) ccw
  arc A199 (29.143, 77.7706) -> (27.94, 78.359) centre (27.94, 76.835) ccw
  arc A200 (27.94, 74.803) -> (26.379, 75.5341) centre (27.94, 76.835) cw
  arc A201 (29.7329, 75.8788) -> (27.94, 74.803) centre (27.9399, 76.835) cw
  arc A202 (27.94, 78.867) -> (26.3888, 78.1476) centre (27.94, 76.835) ccw
  arc A203 (29.7043, 77.8432) -> (27.94, 78.867) centre (27.9401, 76.835) ccw
  line L6009 (36.52, 58.32) -> (36.52, 71.07)
  line L6010 (36.52, 71.07) -> (4.02, 71.07)
  line L6011 (4.02, 71.07) -> (4.02, 58.32)
  line L6012 (4.02, 58.32) -> (36.52, 58.32)
  arc A204 (18.77, 64.695) -> (21.77, 64.695) centre (20.27, 64.695) ccw
  arc A205 (21.77, 64.695) -> (18.77, 64.695) centre (20.27, 64.695) ccw
  line L6013 (63.81, 71.22) -> (63.81, 58.47)
  line L6014 (63.81, 58.47) -> (96.31, 58.47)
  line L6015 (96.31, 58.47) -> (96.31, 71.22)
  line L6016 (96.31, 71.22) -> (63.81, 71.22)
  arc A206 (78.56, 64.845) -> (81.56, 64.845) centre (80.06, 64.845) ccw
  arc A207 (81.56, 64.845) -> (78.56, 64.845) centre (80.06, 64.845) ccw
  line L6017 (10.143, 54.229) -> (1.143, 54.229)
  line L6018 (1.143, 54.229) -> (1.143, 32.229)
  line L6019 (1.143, 32.229) -> (10.143, 32.229)
  line L6020 (10.143, 32.229) -> (10.143, 54.229)
  arc A208 (4.143, 43.229) -> (7.143, 43.229) centre (5.643, 43.229) ccw
  arc A209 (7.143, 43.229) -> (4.143, 43.229) centre (5.643, 43.229) ccw
  line L6021 (22.843, 54.229) -> (13.843, 54.229)
  line L6022 (13.843, 54.229) -> (13.843, 32.229)
  line L6023 (13.843, 32.229) -> (22.843, 32.229)
  line L6024 (22.843, 32.229) -> (22.843, 54.229)
  arc A210 (19.843, 43.229) -> (16.843, 43.229) centre (18.343, 43.229) ccw
  arc A211 (16.843, 43.229) -> (19.843, 43.229) centre (18.343, 43.229) ccw
  line L6025 (35.543, 54.229) -> (26.543, 54.229)
  line L6026 (26.543, 54.229) -> (26.543, 32.229)
  line L6027 (26.543, 32.229) -> (35.543, 32.229)
  line L6028 (35.543, 32.229) -> (35.543, 54.229)
  arc A212 (29.543, 43.229) -> (32.543, 43.229) centre (31.043, 43.229) ccw
  arc A213 (32.543, 43.229) -> (29.543, 43.229) centre (31.043, 43.229) ccw
  line L6029 (48.243, 54.229) -> (39.243, 54.229)
  line L6030 (39.243, 54.229) -> (39.243, 32.229)
  line L6031 (39.243, 32.229) -> (48.243, 32.229)
  line L6032 (48.243, 32.229) -> (48.243, 54.229)
  arc A214 (42.243, 43.229) -> (45.243, 43.229) centre (43.743, 43.229) ccw
  arc A215 (45.243, 43.229) -> (42.243, 43.229) centre (43.743, 43.229) ccw
  line L6033 (61.578, 54.229) -> (52.578, 54.229)
  line L6034 (52.578, 54.229) -> (52.578, 32.229)
  line L6035 (52.578, 32.229) -> (61.578, 32.229)
  line L6036 (61.578, 32.229) -> (61.578, 54.229)
  arc A216 (58.578, 43.229) -> (55.578, 43.229) centre (57.078, 43.229) ccw
  arc A217 (55.578, 43.229) -> (58.578, 43.229) centre (57.078, 43.229) ccw
  line L6037 (74.278, 54.229) -> (65.278, 54.229)
  line L6038 (65.278, 54.229) -> (65.278, 32.229)
  line L6039 (65.278, 32.229) -> (74.278, 32.229)
  line L6040 (74.278, 32.229) -> (74.278, 54.229)
  arc A218 (71.278, 43.229) -> (68.278, 43.229) centre (69.778, 43.229) ccw
  arc A219 (68.278, 43.229) -> (71.278, 43.229) centre (69.778, 43.229) ccw
  line L6041 (86.978, 54.229) -> (77.978, 54.229)
  line L6042 (77.978, 54.229) -> (77.978, 32.229)
  line L6043 (77.978, 32.229) -> (86.978, 32.229)
  line L6044 (86.978, 32.229) -> (86.978, 54.229)
  arc A220 (83.978, 43.229) -> (80.978, 43.229) centre (82.478, 43.229) ccw
  arc A221 (80.978, 43.229) -> (83.978, 43.229) centre (82.478, 43.229) ccw
  line L6045 (99.043, 54.229) -> (90.043, 54.229)
  line L6046 (90.043, 54.229) -> (90.043, 32.229)
  line L6047 (90.043, 32.229) -> (99.043, 32.229)
  line L6048 (99.043, 32.229) -> (99.043, 54.229)
  arc A222 (96.043, 43.229) -> (93.043, 43.229) centre (94.543, 43.229) ccw
  arc A223 (93.043, 43.229) -> (96.043, 43.229) centre (94.543, 43.229) ccw
  line L6049 (50.8, 79.375) -> (50.8, 71.375)
  line L6050 (55.88, 79.375) -> (50.8, 79.375)
  line L6051 (50.8, 79.375) -> (45.72, 79.375)
  line L6052 (45.72, 79.375) -> (45.72, 78.74)
  line L6053 (45.72, 78.74) -> (45.72, 72.0725)
  line L6054 (45.72, 72.0725) -> (45.72, 71.375)
  line L6055 (45.72, 71.375) -> (50.8, 71.375)
  line L6056 (50.8, 71.375) -> (55.88, 71.375)
  line L6057 (55.88, 71.375) -> (55.88, 72.0725)
  line L6058 (55.88, 72.0725) -> (55.88, 72.263)
  line L6059 (55.88, 72.263) -> (55.88, 73.025)
  line L6060 (55.88, 73.025) -> (55.88, 78.74)
  line L6061 (55.88, 78.74) -> (55.88, 79.375)
  line L6062 (55.88, 72.0725) -> (45.72, 72.0725)
  line L6063 (55.88, 72.263) -> (56.388, 71.755)
  line L6064 (56.388, 71.755) -> (56.388, 73.533)
  line L6065 (56.388, 73.533) -> (55.88, 73.025)
  line L6066 (55.88, 78.74) -> (45.72, 78.74)
  arc A224 (49.86, 75.375) -> (46.66, 75.375) centre (48.26, 75.375) ccw
  arc A225 (46.66, 75.375) -> (49.86, 75.375) centre (48.26, 75.375) ccw
  arc A226 (54.94, 75.375) -> (51.74, 75.375) centre (53.34, 75.375) ccw
  arc A227 (51.74, 75.375) -> (54.94, 75.375) centre (53.34, 75.375) ccw
  line L6067 (0.635, 13.335) -> (8.635, 13.335)
  line L6068 (0.635, 18.415) -> (0.635, 13.335)
  line L6069 (0.635, 13.335) -> (0.635, 8.255)
  line L6070 (0.635, 8.255) -> (1.27, 8.255)
  line L6071 (1.27, 8.255) -> (7.9375, 8.255)
  line L6072 (7.9375, 8.255) -> (8.635, 8.255)
  line L6073 (8.635, 8.255) -> (8.635, 13.335)
  line L6074 (8.635, 13.335) -> (8.635, 18.415)
  line L6075 (8.635, 18.415) -> (7.9375, 18.415)
  line L6076 (7.9375, 18.415) -> (7.747, 18.415)
  line L6077 (7.747, 18.415) -> (6.985, 18.415)
  line L6078 (6.985, 18.415) -> (1.27, 18.415)
  line L6079 (1.27, 18.415) -> (0.635, 18.415)
  line L6080 (7.9375, 18.415) -> (7.9375, 8.255)
  line L6081 (7.747, 18.415) -> (8.255, 18.923)
  line L6082 (8.255, 18.923) -> (6.477, 18.923)
  line L6083 (6.477, 18.923) -> (6.985, 18.415)
  line L6084 (1.27, 18.415) -> (1.27, 8.255)
  line L6085 (6.235, 10.795) -> (6.235, 10.795)
  arc A228 (3.035, 10.795) -> (6.235, 10.795) centre (4.635, 10.795) ccw
  arc A229 (6.235, 10.795) -> (3.035, 10.795) centre (4.635, 10.795) ccw
  arc A230 (6.235, 15.875) -> (3.035, 15.875) centre (4.635, 15.875) ccw
  arc A231 (3.035, 15.875) -> (6.235, 15.875) centre (4.635, 15.875) ccw
  line L6086 (6.235, 15.875) -> (6.235, 15.875)
  line L6087 (18.415, 8.89) -> (18.415, 0.89)
  line L6088 (23.495, 8.89) -> (18.415, 8.89)
  line L6089 (18.415, 8.89) -> (13.335, 8.89)
  line L6090 (13.335, 8.89) -> (13.335, 8.255)
  line L6091 (13.335, 8.255) -> (13.335, 1.5875)
  line L6092 (13.335, 1.5875) -> (13.335, 0.89)
  line L6093 (13.335, 0.89) -> (18.415, 0.89)
  line L6094 (18.415, 0.89) -> (23.495, 0.89)
  line L6095 (23.495, 0.89) -> (23.495, 1.5875)
  line L6096 (23.495, 1.5875) -> (23.495, 1.778)
  line L6097 (23.495, 1.778) -> (23.495, 2.54)
  line L6098 (23.495, 2.54) -> (23.495, 8.255)
  line L6099 (23.495, 8.255) -> (23.495, 8.89)
  line L6100 (23.495, 1.5875) -> (13.335, 1.5875)
  line L6101 (23.495, 1.778) -> (24.003, 1.27)
  line L6102 (24.003, 1.27) -> (24.003, 3.048)
  line L6103 (24.003, 3.048) -> (23.495, 2.54)
  line L6104 (23.495, 8.255) -> (13.335, 8.255)
  arc A232 (17.475, 4.89) -> (14.275, 4.89) centre (15.875, 4.89) ccw
  arc A233 (14.275, 4.89) -> (17.475, 4.89) centre (15.875, 4.89) ccw
  arc A234 (19.355, 4.89) -> (22.555, 4.89) centre (20.955, 4.89) ccw
  line L6105 (22.555, 4.89) -> (22.555, 4.89)
  arc A235 (22.555, 4.89) -> (19.355, 4.89) centre (20.955, 4.89) ccw
  line L6106 (31.115, 8.89) -> (31.115, 0.89)
  line L6107 (36.195, 8.89) -> (31.115, 8.89)
  line L6108 (31.115, 8.89) -> (26.035, 8.89)
  line L6109 (26.035, 8.89) -> (26.035, 8.255)
  line L6110 (26.035, 8.255) -> (26.035, 1.5875)
  line L6111 (26.035, 1.5875) -> (26.035, 0.89)
  line L6112 (26.035, 0.89) -> (31.115, 0.89)
  line L6113 (31.115, 0.89) -> (36.195, 0.89)
  line L6114 (36.195, 0.89) -> (36.195, 1.5875)
  line L6115 (36.195, 1.5875) -> (36.195, 1.778)
  line L6116 (36.195, 1.778) -> (36.195, 2.54)
  line L6117 (36.195, 2.54) -> (36.195, 8.255)
  line L6118 (36.195, 8.255) -> (36.195, 8.89)
  line L6119 (36.195, 1.5875) -> (26.035, 1.5875)
  line L6120 (36.195, 1.778) -> (36.703, 1.27)
  line L6121 (36.703, 1.27) -> (36.703, 3.048)
  line L6122 (36.703, 3.048) -> (36.195, 2.54)
  line L6123 (36.195, 8.255) -> (26.035, 8.255)
  arc A236 (26.975, 4.89) -> (30.175, 4.89) centre (28.575, 4.89) ccw
  line L6124 (30.175, 4.89) -> (30.175, 4.89)
  arc A237 (30.175, 4.89) -> (26.975, 4.89) centre (28.575, 4.89) ccw
  arc A238 (35.255, 4.89) -> (32.055, 4.89) centre (33.655, 4.89) ccw
  arc A239 (32.055, 4.89) -> (35.255, 4.89) centre (33.655, 4.89) ccw
  line L6125 (43.815, 8.89) -> (43.815, 0.89)
  line L6126 (48.895, 8.89) -> (43.815, 8.89)
  line L6127 (43.815, 8.89) -> (38.735, 8.89)
  line L6128 (38.735, 8.89) -> (38.735, 8.255)
  line L6129 (38.735, 8.255) -> (38.735, 1.5875)
  line L6130 (38.735, 1.5875) -> (38.735, 0.89)
  line L6131 (38.735, 0.89) -> (43.815, 0.89)
  line L6132 (43.815, 0.89) -> (48.895, 0.89)
  line L6133 (48.895, 0.89) -> (48.895, 1.5875)
  line L6134 (48.895, 1.5875) -> (48.895, 1.778)
  line L6135 (48.895, 1.778) -> (48.895, 2.54)
  line L6136 (48.895, 2.54) -> (48.895, 8.255)
  line L6137 (48.895, 8.255) -> (48.895, 8.89)
  line L6138 (48.895, 1.5875) -> (38.735, 1.5875)
  line L6139 (48.895, 1.778) -> (49.403, 1.27)
  line L6140 (49.403, 1.27) -> (49.403, 3.048)
  line L6141 (49.403, 3.048) -> (48.895, 2.54)
  line L6142 (48.895, 8.255) -> (38.735, 8.255)
  arc A240 (39.675, 4.89) -> (42.875, 4.89) centre (41.275, 4.89) ccw
  arc A241 (42.875, 4.89) -> (39.675, 4.89) centre (41.275, 4.89) ccw
  arc A242 (47.955, 4.89) -> (44.755, 4.89) centre (46.355, 4.89) ccw
  arc A243 (44.755, 4.89) -> (47.955, 4.89) centre (46.355, 4.89) ccw
  line L6143 (57.15, 8.89) -> (57.15, 0.89)
  line L6144 (62.23, 8.89) -> (57.15, 8.89)
  line L6145 (57.15, 8.89) -> (52.07, 8.89)
  line L6146 (52.07, 8.89) -> (52.07, 8.255)
  line L6147 (52.07, 8.255) -> (52.07, 1.5875)
  line L6148 (52.07, 1.5875) -> (52.07, 0.89)
  line L6149 (52.07, 0.89) -> (57.15, 0.89)
  line L6150 (57.15, 0.89) -> (62.23, 0.89)
  line L6151 (62.23, 0.89) -> (62.23, 1.5875)
  line L6152 (62.23, 1.5875) -> (62.23, 1.778)
  line L6153 (62.23, 1.778) -> (62.23, 2.54)
  line L6154 (62.23, 2.54) -> (62.23, 8.255)
  line L6155 (62.23, 8.255) -> (62.23, 8.89)
  line L6156 (62.23, 1.5875) -> (52.07, 1.5875)
  line L6157 (62.23, 1.778) -> (62.738, 1.27)
  line L6158 (62.738, 1.27) -> (62.738, 3.048)
  line L6159 (62.738, 3.048) -> (62.23, 2.54)
  line L6160 (62.23, 8.255) -> (52.07, 8.255)
  arc A244 (53.01, 4.89) -> (56.21, 4.89) centre (54.61, 4.89) ccw
  arc A245 (56.21, 4.89) -> (53.01, 4.89) centre (54.61, 4.89) ccw
  arc A246 (58.09, 4.89) -> (61.29, 4.89) centre (59.69, 4.89) ccw
  arc A247 (61.29, 4.89) -> (58.09, 4.89) centre (59.69, 4.89) ccw
  line L6161 (69.85, 8.89) -> (69.85, 0.89)
  line L6162 (74.93, 8.89) -> (69.85, 8.89)
  line L6163 (69.85, 8.89) -> (64.77, 8.89)
  line L6164 (64.77, 8.89) -> (64.77, 8.255)
  line L6165 (64.77, 8.255) -> (64.77, 1.5875)
  line L6166 (64.77, 1.5875) -> (64.77, 0.89)
  line L6167 (64.77, 0.89) -> (69.85, 0.89)
  line L6168 (69.85, 0.89) -> (74.93, 0.89)
  line L6169 (74.93, 0.89) -> (74.93, 1.5875)
  line L6170 (74.93, 1.5875) -> (74.93, 1.778)
  line L6171 (74.93, 1.778) -> (74.93, 2.54)
  line L6172 (74.93, 2.54) -> (74.93, 8.255)
  line L6173 (74.93, 8.255) -> (74.93, 8.89)
  line L6174 (74.93, 1.5875) -> (64.77, 1.5875)
  line L6175 (74.93, 1.778) -> (75.438, 1.27)
  line L6176 (75.438, 1.27) -> (75.438, 3.048)
  line L6177 (75.438, 3.048) -> (74.93, 2.54)
  line L6178 (74.93, 8.255) -> (64.77, 8.255)
  arc A248 (65.71, 4.89) -> (68.91, 4.89) centre (67.31, 4.89) ccw
  arc A249 (68.91, 4.89) -> (65.71, 4.89) centre (67.31, 4.89) ccw
  arc A250 (73.99, 4.89) -> (70.79, 4.89) centre (72.39, 4.89) ccw
  arc A251 (70.79, 4.89) -> (73.99, 4.89) centre (72.39, 4.89) ccw
  line L6179 (82.55, 8.89) -> (82.55, 0.89)
  line L6180 (87.63, 8.89) -> (82.55, 8.89)
  line L6181 (82.55, 8.89) -> (77.47, 8.89)
  line L6182 (77.47, 8.89) -> (77.47, 8.255)
  line L6183 (77.47, 8.255) -> (77.47, 1.5875)
  line L6184 (77.47, 1.5875) -> (77.47, 0.89)
  line L6185 (77.47, 0.89) -> (82.55, 0.89)
  line L6186 (82.55, 0.89) -> (87.63, 0.89)
  line L6187 (87.63, 0.89) -> (87.63, 1.5875)
  line L6188 (87.63, 1.5875) -> (87.63, 1.778)
  line L6189 (87.63, 1.778) -> (87.63, 2.54)
  line L6190 (87.63, 2.54) -> (87.63, 8.255)
  line L6191 (87.63, 8.255) -> (87.63, 8.89)
  line L6192 (87.63, 1.5875) -> (77.47, 1.5875)
  line L6193 (87.63, 1.778) -> (88.138, 1.27)
  line L6194 (88.138, 1.27) -> (88.138, 3.048)
  line L6195 (88.138, 3.048) -> (87.63, 2.54)
  line L6196 (87.63, 8.255) -> (77.47, 8.255)
  arc A252 (81.61, 4.89) -> (78.41, 4.89) centre (80.01, 4.89) ccw
  arc A253 (78.41, 4.89) -> (81.61, 4.89) centre (80.01, 4.89) ccw
  arc A254 (86.69, 4.89) -> (83.49, 4.89) centre (85.09, 4.89) ccw
  arc A255 (83.49, 4.89) -> (86.69, 4.89) centre (85.09, 4.89) ccw
  line L6197 (91.44, 13.335) -> (99.44, 13.335)
  line L6198 (91.44, 18.415) -> (91.44, 13.335)
  line L6199 (91.44, 13.335) -> (91.44, 8.255)
  line L6200 (91.44, 8.255) -> (92.075, 8.255)
  line L6201 (92.075, 8.255) -> (98.7425, 8.255)
  line L6202 (98.7425, 8.255) -> (99.44, 8.255)
  line L6203 (99.44, 8.255) -> (99.44, 13.335)
  line L6204 (99.44, 13.335) -> (99.44, 18.415)
  line L6205 (99.44, 18.415) -> (98.7425, 18.415)
  line L6206 (98.7425, 18.415) -> (98.552, 18.415)
  line L6207 (98.552, 18.415) -> (97.79, 18.415)
  line L6208 (97.79, 18.415) -> (92.075, 18.415)
  line L6209 (92.075, 18.415) -> (91.44, 18.415)
  line L6210 (98.7425, 18.415) -> (98.7425, 8.255)
  line L6211 (98.552, 18.415) -> (99.06, 18.923)
  line L6212 (99.06, 18.923) -> (97.282, 18.923)
  line L6213 (97.282, 18.923) -> (97.79, 18.415)
  line L6214 (92.075, 18.415) -> (92.075, 8.255)
  arc A256 (93.84, 10.795) -> (97.04, 10.795) centre (95.44, 10.795) ccw
  arc A257 (97.04, 10.795) -> (93.84, 10.795) centre (95.44, 10.795) ccw
  arc A258 (97.04, 15.875) -> (93.84, 15.875) centre (95.44, 15.875) ccw
  arc A259 (93.84, 15.875) -> (97.04, 15.875) centre (95.44, 15.875) ccw
  arc A260 (22.86, 78.359) -> (24.1001, 77.7208) centre (22.86, 76.835) cw
  arc A261 (21.6408, 77.7494) -> (22.86, 78.359) centre (22.86, 76.835) cw
  arc A262 (22.86, 75.311) -> (24.063, 75.8994) centre (22.86, 76.835) ccw
  arc A263 (21.657, 75.8994) -> (22.86, 75.311) centre (22.86, 76.835) ccw
  arc A264 (22.86, 78.867) -> (24.421, 78.1359) centre (22.86, 76.835) cw
  arc A265 (21.0671, 77.7912) -> (22.86, 78.867) centre (22.8601, 76.835) cw
  arc A266 (22.86, 74.803) -> (24.4112, 75.5224) centre (22.86, 76.835) ccw
  arc A267 (21.0957, 75.8268) -> (22.86, 74.803) centre (22.8599, 76.835) ccw
  arc A268 (77.47, 74.676) -> (76.2299, 75.3142) centre (77.47, 76.2) cw
  arc A269 (78.6892, 75.2856) -> (77.47, 74.676) centre (77.47, 76.2) cw
  arc A270 (77.47, 77.724) -> (76.267, 77.1356) centre (77.47, 76.2) ccw
  arc A271 (78.673, 77.1356) -> (77.47, 77.724) centre (77.47, 76.2) ccw
  arc A272 (77.47, 74.168) -> (75.909, 74.8991) centre (77.47, 76.2) cw
  arc A273 (79.2629, 75.2438) -> (77.47, 74.168) centre (77.4699, 76.2) cw
  arc A274 (77.47, 78.232) -> (75.9188, 77.5126) centre (77.47, 76.2) ccw
  arc A275 (79.2343, 77.2082) -> (77.47, 78.232) centre (77.4701, 76.2) ccw
  arc A276 (11.43, 18.034) -> (12.6701, 17.3958) centre (11.43, 16.51) cw
  arc A277 (10.2108, 17.4244) -> (11.43, 18.034) centre (11.43, 16.51) cw
  arc A278 (11.43, 14.986) -> (12.633, 15.5744) centre (11.43, 16.51) ccw
  arc A279 (10.227, 15.5744) -> (11.43, 14.986) centre (11.43, 16.51) ccw
  arc A280 (11.43, 18.542) -> (12.991, 17.8109) centre (11.43, 16.51) cw
  arc A281 (9.6371, 17.4662) -> (11.43, 18.542) centre (11.4301, 16.51) cw
  arc A282 (11.43, 14.478) -> (12.9812, 15.1974) centre (11.43, 16.51) ccw
  arc A283 (9.6657, 15.5018) -> (11.43, 14.478) centre (11.4299, 16.51) ccw
  arc A284 (77.47, 14.986) -> (76.2299, 15.6242) centre (77.47, 16.51) cw
  arc A285 (78.6892, 15.5956) -> (77.47, 14.986) centre (77.47, 16.51) cw
  arc A286 (77.47, 18.034) -> (76.267, 17.4456) centre (77.47, 16.51) ccw
  arc A287 (78.673, 17.4456) -> (77.47, 18.034) centre (77.47, 16.51) ccw
  arc A288 (77.47, 14.478) -> (75.909, 15.2091) centre (77.47, 16.51) cw
  arc A289 (79.2629, 15.5538) -> (77.47, 14.478) centre (77.4699, 16.51) cw
  arc A290 (77.47, 18.542) -> (75.9188, 17.8226) centre (77.47, 16.51) ccw
  arc A291 (79.2343, 17.5182) -> (77.47, 18.542) centre (77.4701, 16.51) ccw
  arc A292 (66.04, 14.986) -> (64.7999, 15.6242) centre (66.04, 16.51) cw
  arc A293 (67.2592, 15.5956) -> (66.04, 14.986) centre (66.04, 16.51) cw
  arc A294 (66.04, 18.034) -> (64.837, 17.4456) centre (66.04, 16.51) ccw
  arc A295 (67.243, 17.4456) -> (66.04, 18.034) centre (66.04, 16.51) ccw
  arc A296 (66.04, 14.478) -> (64.479, 15.2091) centre (66.04, 16.51) cw
  arc A297 (67.8329, 15.5538) -> (66.04, 14.478) centre (66.0399, 16.51) cw
  arc A298 (66.04, 18.542) -> (64.4888, 17.8226) centre (66.04, 16.51) ccw
  arc A299 (67.8043, 17.5182) -> (66.04, 18.542) centre (66.0401, 16.51) ccw
  arc A300 (55.88, 14.986) -> (54.6399, 15.6242) centre (55.88, 16.51) cw
  arc A301 (57.0992, 15.5956) -> (55.88, 14.986) centre (55.88, 16.51) cw
  arc A302 (55.88, 18.034) -> (54.677, 17.4456) centre (55.88, 16.51) ccw
  arc A303 (57.083, 17.4456) -> (55.88, 18.034) centre (55.88, 16.51) ccw
  arc A304 (55.88, 14.478) -> (54.319, 15.2091) centre (55.88, 16.51) cw
  arc A305 (57.6729, 15.5538) -> (55.88, 14.478) centre (55.8799, 16.51) cw
  arc A306 (55.88, 18.542) -> (54.3288, 17.8226) centre (55.88, 16.51) ccw
  arc A307 (57.6443, 17.5182) -> (55.88, 18.542) centre (55.8801, 16.51) ccw
  arc A308 (47.625, 18.034) -> (48.8651, 17.3958) centre (47.625, 16.51) cw
  arc A309 (46.4058, 17.4244) -> (47.625, 18.034) centre (47.625, 16.51) cw
  arc A310 (47.625, 14.986) -> (48.828, 15.5744) centre (47.625, 16.51) ccw
  arc A311 (46.422, 15.5744) -> (47.625, 14.986) centre (47.625, 16.51) ccw
  arc A312 (47.625, 18.542) -> (49.186, 17.8109) centre (47.625, 16.51) cw
  arc A313 (45.8321, 17.4662) -> (47.625, 18.542) centre (47.6251, 16.51) cw
  arc A314 (47.625, 14.478) -> (49.1762, 15.1974) centre (47.625, 16.51) ccw
  arc A315 (45.8607, 15.5018) -> (47.625, 14.478) centre (47.6249, 16.51) ccw
  arc A316 (36.83, 18.034) -> (38.0701, 17.3958) centre (36.83, 16.51) cw
  arc A317 (35.6108, 17.4244) -> (36.83, 18.034) centre (36.83, 16.51) cw
  arc A318 (36.83, 14.986) -> (38.033, 15.5744) centre (36.83, 16.51) ccw
  arc A319 (35.627, 15.5744) -> (36.83, 14.986) centre (36.83, 16.51) ccw
  arc A320 (36.83, 18.542) -> (38.391, 17.8109) centre (36.83, 16.51) cw
  arc A321 (35.0371, 17.4662) -> (36.83, 18.542) centre (36.8301, 16.51) cw
  arc A322 (36.83, 14.478) -> (38.3812, 15.1974) centre (36.83, 16.51) ccw
  arc A323 (35.0657, 15.5018) -> (36.83, 14.478) centre (36.8299, 16.51) ccw
  arc A324 (24.13, 18.034) -> (25.3701, 17.3958) centre (24.13, 16.51) cw
  arc A325 (22.9108, 17.4244) -> (24.13, 18.034) centre (24.13, 16.51) cw
  arc A326 (24.13, 14.986) -> (25.333, 15.5744) centre (24.13, 16.51) ccw
  arc A327 (22.927, 15.5744) -> (24.13, 14.986) centre (24.13, 16.51) ccw
  arc A328 (24.13, 18.542) -> (25.691, 17.8109) centre (24.13, 16.51) cw
  arc A329 (22.3371, 17.4662) -> (24.13, 18.542) centre (24.1301, 16.51) cw
  arc A330 (24.13, 14.478) -> (25.6812, 15.1974) centre (24.13, 16.51) ccw
  arc A331 (22.3657, 15.5018) -> (24.13, 14.478) centre (24.1299, 16.51) ccw
  arc A332 (88.9, 14.986) -> (87.6599, 15.6242) centre (88.9, 16.51) cw
  arc A333 (90.1192, 15.5956) -> (88.9, 14.986) centre (88.9, 16.51) cw
  arc A334 (88.9, 18.034) -> (87.697, 17.4456) centre (88.9, 16.51) ccw
  arc A335 (90.103, 17.4456) -> (88.9, 18.034) centre (88.9, 16.51) ccw
  arc A336 (88.9, 14.478) -> (87.339, 15.2091) centre (88.9, 16.51) cw
  arc A337 (90.6929, 15.5538) -> (88.9, 14.478) centre (88.8999, 16.51) cw
  arc A338 (88.9, 18.542) -> (87.3488, 17.8226) centre (88.9, 16.51) ccw
  arc A339 (90.6643, 17.5182) -> (88.9, 18.542) centre (88.9001, 16.51) ccw
  arc A340 (17.145, 75.946) -> (16.891, 75.692) centre (16.891, 75.946) cw
  arc A341 (17.145, 77.724) -> (16.891, 77.978) centre (16.891, 77.724) ccw
  arc A342 (11.049, 77.978) -> (10.795, 77.724) centre (11.049, 77.724) ccw
  arc A343 (11.049, 75.692) -> (10.795, 75.946) centre (11.049, 75.946) cw
  line L6215 (17.145, 77.724) -> (17.145, 75.946)
  line L6216 (16.891, 75.692) -> (16.51, 75.692)
  line L6217 (16.383, 75.819) -> (16.51, 75.692)
  line L6218 (16.891, 77.978) -> (16.51, 77.978)
  line L6219 (16.383, 77.851) -> (16.51, 77.978)
  line L6220 (11.557, 75.819) -> (11.43, 75.692)
  line L6221 (11.557, 75.819) -> (16.383, 75.819)
  line L6222 (11.557, 77.851) -> (11.43, 77.978)
  line L6223 (11.557, 77.851) -> (16.383, 77.851)
  line L6224 (11.049, 75.692) -> (11.43, 75.692)
  line L6225 (11.049, 77.978) -> (11.43, 77.978)
  line L6226 (10.795, 77.724) -> (10.795, 75.946)
  line L6227 (10.795, 76.5302) -> (10.795, 77.1398)
  line L6228 (9.9314, 77.1398) -> (9.9314, 76.5302)
  line L6229 (10.795, 77.1398) -> (9.9314, 77.1398)
  line L6230 (9.9314, 76.5302) -> (10.795, 76.5302)
  line L6231 (18.0086, 76.5302) -> (18.0086, 77.1398)
  line L6232 (18.0086, 77.1398) -> (17.145, 77.1398)
  line L6233 (17.145, 76.5302) -> (18.0086, 76.5302)
  line L6234 (17.145, 77.1398) -> (17.145, 76.5302)
  arc A344 (83.185, 77.089) -> (83.439, 77.343) centre (83.439, 77.089) cw
  arc A345 (83.185, 75.311) -> (83.439, 75.057) centre (83.439, 75.311) ccw
  arc A346 (89.281, 75.057) -> (89.535, 75.311) centre (89.281, 75.311) ccw
  arc A347 (89.281, 77.343) -> (89.535, 77.089) centre (89.281, 77.089) cw
  line L6235 (83.185, 75.311) -> (83.185, 77.089)
  line L6236 (83.439, 77.343) -> (83.82, 77.343)
  line L6237 (83.947, 77.216) -> (83.82, 77.343)
  line L6238 (83.439, 75.057) -> (83.82, 75.057)
  line L6239 (83.947, 75.184) -> (83.82, 75.057)
  line L6240 (88.773, 77.216) -> (88.9, 77.343)
  line L6241 (88.773, 77.216) -> (83.947, 77.216)
  line L6242 (88.773, 75.184) -> (88.9, 75.057)
  line L6243 (88.773, 75.184) -> (83.947, 75.184)
  line L6244 (89.281, 77.343) -> (88.9, 77.343)
  line L6245 (89.281, 75.057) -> (88.9, 75.057)
  line L6246 (89.535, 75.311) -> (89.535, 77.089)
  line L6247 (90.3986, 76.5048) -> (89.535, 76.5048)
  line L6248 (89.535, 75.8952) -> (90.3986, 75.8952)
  line L6249 (89.535, 76.5048) -> (89.535, 75.8952)
  line L6250 (90.3986, 75.8952) -> (90.3986, 76.5048)
  line L6251 (82.3214, 75.8952) -> (83.185, 75.8952)
  line L6252 (83.185, 75.8952) -> (83.185, 76.5048)
  line L6253 (83.185, 76.5048) -> (82.3214, 76.5048)
  line L6254 (82.3214, 76.5048) -> (82.3214, 75.8952)
  arc A348 (9.271, 22.225) -> (9.017, 22.479) centre (9.271, 22.479) cw
  arc A349 (11.049, 22.225) -> (11.303, 22.479) centre (11.049, 22.479) ccw